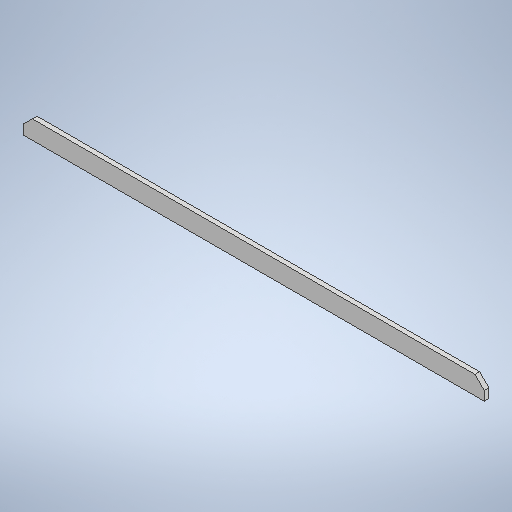
# Autodesk Inventor part: vslot hinge brace top
Saved by Autodesk Inventor 2025 (Build 290162010, 162A)
## iProperties
Created: 2024-06-18
Part Number: vslot hinge brace top
Material: Generic
Document SubType Name: Modeling
Designer: Alan Thomas
Mass: 393.2 g
Surface Area: 990.657 cm^2
Volume: 393.2 cm^3
Density: 1 g/cm^3
Appearance: Default
Author: Alan Thomas
Autodesk Inventor part; units mm, degrees
ref_plane "YZ Plane" through (0, 0, 0) normal (1, 0, 0) x (0, 1, 0)
ref_plane "XZ Plane" through (0, 0, 0) normal (0, 1, 0) x (-1, 0, 0)
ref_plane "XY Plane" through (0, 0, 0) normal (0, 0, 1) x (1, 0, 0)
sketch "Sketch1" plane through (0, 0, 0) normal (0, 0, 1) x (1, 0, 0)
  line L0 (0, 0) -> (993, 0)
  line L1 (993, 0) -> (993, 40)
  line L2 (993, 40) -> (0, 40)
  line L3 (0, 40) -> (0, 0)
  dimension "d0" = 993
  dimension "d1" = 40
  constraints: 8 end point, 2 parallel, 1 horizontal, 1 perpendicular
  measures "d0" distance of L2.end L1.end
  measures "d1" distance of L1.end L0.end
extrude "Extrusion1" add sketch "Sketch1" along normal blind 10
sketch "Sketch5" plane through (0, 0, 10) normal (0, 0, 1) x (1, 0, 0)
  line L0 (0, 40) -> (0, 0) projected
  line L1 (0, 20) -> (20.0002, 40)
  line L2 (993, 40) -> (0, 40) projected
  line L3 (993, 0) -> (993, 40) projected
  line L4 (993, 20) -> (973.0002, 40)
  constraints: 4 end point, 2 midpoint, 1 perpendicular, 1 point on line
extrude "Extrusion5" cut sketch "Sketch5" against normal blind 10
body "Solid1"
